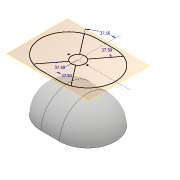
# Autodesk Inventor part: Part12
Saved by Autodesk Inventor 2018 (Build 220112000, 112)
## iProperties
Created: 2017-05-23
Part Number: Part12
Material: Generic
Document SubType Name: Modeling
Designer: anand
Density: 1 g/cm^3
Appearance: Default
Author: anand
Autodesk Inventor part; units mm, degrees
ref_plane "YZ Plane" through (0, 0, 0) normal (1, 0, 0) x (0, 1, 0)
ref_plane "XZ Plane" through (0, 0, 0) normal (0, 1, 0) x (-1, 0, 0)
sketch "Sketch1" plane through (0, 0, 0) normal (0, 0, 1) x (1, 0, 0)
  arc A0 (-12.5, 37.1548) -> (-49.9984, 0) centre (-12.5, -0.3452) ccw
  arc A1 (49.9984, 0) -> (12.5, 37.1548) centre (12.5, -0.3452) ccw
  line L0 (-12.5, 37.1548) -> (12.5, 37.1548)
  line L1 (-49.9984, 0) -> (49.9984, 0)
  point P0 (0, 0)
  dimension "d0" = 25
  dimension "d1" = 75
  dimension "d3" = 12.5
  constraints: 4 end point, 4 point on circle, 2 centre point, 2 horizontal, 1 equal radius, 1 horizontal alignment, 1 midpoint, 1 tangent
  measures "d0" distance of A0.centre A1.centre
  measures "d1" diameter of A1
  measures "d3" horizontal distance of point (0, 0) A1.centre
revolve "Revolution1" add sketch "Sketch1" angle 180 about axis through (-49.9984, 0, 0) along (1, 0, 0)
ref_plane "Work Plane2" through (0, 0, 70) normal (0, 0, 1) x (1, 0, 0)
sketch "Sketch3" plane through (0, 0, 70) normal (0, 0, 1) x (1, 0, 0)
  arc A0 (-49.9984, 0) -> (-12.5, -37.1548) centre (-12.5, 0.3452) ccw
  circle A1 centre (0, 0) radius 9.0115
  line L0 (-4.4971, -7.8092) -> (-25.2895, -34.9065)
  line L1 (4.4971, -7.8092) -> (25.2895, -34.9065)
  arc A2 (12.5, -37.1548) -> (49.9984, 0) centre (12.5, 0.3452) ccw
  line L2 (12.5, -37.1548) -> (-12.5, -37.1548)
  line L3 (0, 0) -> (71.363, 0) construction
  arc A3 (-12.5, 37.1548) -> (-49.9984, 0) centre (-12.5, -0.3452) ccw
  line L4 (12.5, 37.1548) -> (-12.5, 37.1548)
  arc A4 (49.9984, 0) -> (12.5, 37.1548) centre (12.5, -0.3452) ccw
  line L5 (-5.348, 7.253) -> (-26.2795, 34.5314)
  line L6 (5.348, 7.253) -> (26.2795, 34.5314)
  line L7 (0, 0) -> (0, 56.6524) construction
  dimension "d14" = 37.5
  dimension "d15" = 37.5
  dimension "d16" = 37.5
  dimension "d17" = 37.5
  constraints: 16 end point, 16 point on circle, 5 centre point, 2 equal length, 1 coincident, 1 horizontal, 1 vertical
  measures "d14" angle of L7 L6
  measures "d15" angle of L7 L5
  measures "d16" angle of L1 L7
  measures "d17" angle of L0 L7
body "Solid1"
